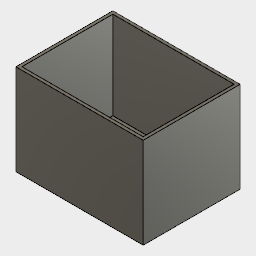
SSD1306_OLED_Box (Autodesk Fusion 360 design; units mm, degrees)
Autodesk Fusion 360 part; units mm, degrees
sketch "Sketch1" plane through (0, 0, 0) normal (0, 1, 0) x (1, 0, 0)
  line L0 (-21, 16) -> (21, 16)
  line L1 (21, 16) -> (21, -16)
  line L2 (21, -16) -> (-21, -16)
  line L3 (-21, -16) -> (-21, 16)
  line L4 (-21, 16) -> (21, -16) construction
  line L5 (21, 16) -> (-21, -16) construction
  dimension "d1" = 42
  dimension "d2" = 32
  constraint perpendicular L0 L1
  constraint parallel L0 L2
  constraint parallel L1 L3
  constraint horizontal L0
  constraint coincident L4 origin
  constraint coincident L5 origin
extrude "Extrude1" add sketch "Sketch1" along normal blind 30
sketch "Sketch2" plane through (0, 30, 0) normal (0, 1, 0) x (-1, 0, 0)
  line L0 (21, 16) -> (-21, 16)
  line L1 (-21, 16) -> (-21, -16)
  line L2 (-21, -16) -> (21, -16)
  line L3 (21, -16) -> (21, 16)
  line L4 (20, -15) -> (-20, -15)
  line L5 (-20, -15) -> (-20, 15)
  line L6 (-20, 15) -> (20, 15)
  line L7 (20, 15) -> (20, -15)
  line L8 (20, -15) -> (-20, 15) construction
  line L9 (-20, -15) -> (20, 15) construction
  dimension "d5" = 40
  dimension "d6" = 30
  constraint perpendicular L4 L5
  constraint parallel L4 L6
  constraint parallel L5 L7
  constraint horizontal L4
  constraint coincident L8 origin
  constraint coincident L9 origin
extrude "Extrude2" cut sketch "Sketch2" against normal blind 29 contours L4 L5 L6 L7
sketch "Sketch3" plane through (0, 1, 0) normal (0, 1, 0) x (-1, 0, 0)
  line L0 (20, 15) -> (-20, 15)
  line L1 (-20, 15) -> (-20, -15)
  line L2 (-20, -15) -> (20, -15)
  line L3 (20, -15) -> (20, 15)
  line L4 (-14, 11) -> (14, 11)
  line L5 (14, 11) -> (14, -11)
  line L6 (14, -11) -> (-14, -11)
  line L7 (-14, -11) -> (-14, 11)
  line L8 (-14, 11) -> (14, -11) construction
  line L9 (14, 11) -> (-14, -11) construction
  dimension "d9" = 28
  dimension "d10" = 22
  constraint perpendicular L4 L5
  constraint parallel L4 L6
  constraint parallel L5 L7
  constraint horizontal L4
  constraint coincident L8 origin
  constraint coincident L9 origin
extrude "Extrude3" cut sketch "Sketch3" against normal blind 1 contours L4 L5 L6 L7
